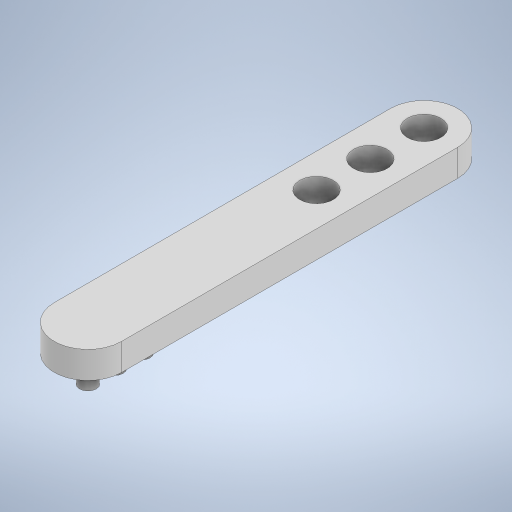
# Autodesk Inventor part: Servo Extension Small
Saved by Autodesk Inventor 2023 (Build 270158000, 158)
## iProperties
Created: 2023-05-02
Part Number: Servo Extension Small
Material: Generic
Document SubType Name: Modeling
Designer: 1senadi
Density: 1 g/cm^3
Appearance: Default
Author: 1senadi
Autodesk Inventor part; units mm, degrees
ref_plane "YZ Plane" through (0, 0, 0) normal (1, 0, 0) x (0, 1, 0)
ref_plane "XZ Plane" through (0, 0, 0) normal (0, 1, 0) x (-1, 0, 0)
ref_plane "XY Plane" through (0, 0, 0) normal (0, 0, 1) x (1, 0, 0)
sketch "Sketch1" plane through (0, 0, 0) normal (0, 1, 0) x (-1, 0, 0)
  circle A0 centre (0, 0) radius 2.5
  line L0 (0, 0) -> (0, -25)
  line L1 (0, 0) -> (25, 0) construction
  circle A1 centre (0, -25) radius 2.5
  line L2 (2.5, -25) -> (2.5, 0)
  line L3 (-2.5, 0) -> (-2.5, -25)
  circle A2 centre (0, -25) radius 1.25
  circle A3 centre (0, -21) radius 1.25
  circle A4 centre (0, -17) radius 1.25
  dimension "d0" = 5
  dimension "d1" = 25
  dimension "d2" = 90
  dimension "d3" = 5
  dimension "d4" = 2.5
  dimension "d7" = 4
  constraints: 8 end point, 5 centre point, 4 point on circle, 3 coincident, 3 vertical, 1 horizontal, 1 perpendicular, 1 tangent, 4 other
  measures "d0" diameter of A0
  measures "d1" distance of L0.start L0.end
  measures "d2" angle of L0 L1
  measures "d3" diameter of A1
  measures "d4" diameter of A2
  measures "d7" distance of A2.centre A3.centre
extrude "Extrusion1" add sketch "Sketch1" along normal blind 2 contours A0 | L2 A1 L0 A3 A4 A0 | A0 L0 A4 A3 A1 L3 | A1
sketch "Sketch2" plane through (0, 0, 0) normal (0, -1, 0) x (1, 0, 0)
  circle A0 centre (0, 0) radius 0.625
  line L0 (2.5, 0) -> (2.5, -25) projected
  circle A1 centre (0, -2) radius 0.625
  circle A2 centre (0, -4) radius 0.625
  dimension "d14" = 1.25
  dimension "d17" = 2
  constraints: 3 centre point, 1 coincident, 1 vertical, 4 other
  measures "d14" diameter of A0
  measures "d17" distance of A0.centre A1.centre
extrude "Extrusion2" add sketch "Sketch2" along normal blind 2
body "Solid1"
